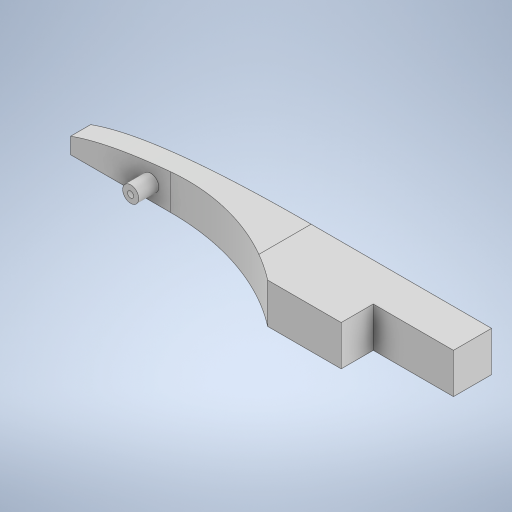
# Autodesk Inventor part: Norma
Saved by Autodesk Inventor 2023 (Build 270158000, 158)
## iProperties
Created: 2023-12-05
Part Number: Norma
Material: Všeobecné
Document SubType Name: Modeling
Designer: clu40164
Mass: 73.9819 g
Surface Area: 163.44 cm^2
Volume: 73.9819 cm^3
Density: 1 g/cm^3
Appearance: Výchozí
Author: clu40164
Autodesk Inventor part; units mm, degrees
ref_plane "YZ Plane" through (0, 0, 0) normal (1, 0, 0) x (0, 1, 0)
ref_plane "XZ Plane" through (0, 0, 0) normal (0, 1, 0) x (-1, 0, 0)
ref_plane "XY Plane" through (0, 0, 0) normal (0, 0, 1) x (1, 0, 0)
sketch "Náčrt1" plane through (0, 0, 0) normal (0, 0, 1) x (1, 0, 0)
  line L0 (0, 0) -> (200, 0)
  line L1 (200, 0) -> (200, 20)
  line L2 (200, 20) -> (110, 20)
  line L3 (0, 0) -> (0, 8)
  line L4 (0, 8) -> (32.9697, 20) construction
  line L5 (32.9697, 20) -> (110, 20) construction
  spline S0 degree 2 poles (0, 8) (32.9697, 20) (110, 20) knots 1 1 1 2 2 2
  dimension "d0" = 200
  dimension "d1" = 20
  dimension "d2" = 90
  dimension "d3" = 8
  dimension "d5" = 160
  constraints: 8 end point, 2 horizontal, 2 perpendicular, 1 vertical, 3 other
  measures "d0" distance of L0.start L0.end
  measures "d1" distance of L0.end L1.end
  measures "d2" distance of L1.end L2.end
  measures "d3" distance of L0.start L3.end
  measures "d5" angle of L5 L4
extrude "Vysunutí1" add sketch "Náčrt1" along normal blind 35
sketch "Náčrt2" plane through (0, 0, 0) normal (0, -1, 0) x (1, 0, 0)
  line L0 (0, 0) -> (0, 35) projected
  line L1 (0, 10) -> (50, 10)
  arc A0 (50, 10) -> (123.3144, 35) centre (50, 130) ccw
  line L2 (160, 35) -> (160, 19)
  line L3 (160, 19) -> (200, 19)
  line L4 (200, 0) -> (200, 35) projected
  line L5 (0, 35) -> (200, 35) projected
  line L6 (160, 35) -> (123.3144, 35)
  line L7 (200, 19) -> (200, 0)
  line L8 (0, 0) -> (200, 0) projected
  line L9 (0, 0) -> (0, 10)
  line L10 (0, 0) -> (200, 0)
  dimension "d8" = 50
  dimension "d9" = 240
  dimension "d11" = 16
  dimension "d12" = 40
  dimension "d13" = 10
  constraints: 14 end point, 5 perpendicular, 2 point on circle, 2 point on line, 1 centre point, 1 collinear, 1 horizontal, 1 horizontal alignment, 1 tangent, 1 vertical, 1 vertical alignment
  measures "d8" distance of L1.end L1.start
  measures "d9" diameter of A0
  measures "d11" distance of L2.start L2.end
  measures "d12" distance of L2.end L3.end
  measures "d13" distance of L0.start L1.start
extrude "Vysunutí2" cut sketch "Náčrt2" against normal blind 35 contours L0 L1 A0 L5 L2 L3 L4 L8 keep common part
sketch "Náčrt3" plane through (0, 0, 10) normal (0, 0, 1) x (1, 0, 0)
  circle A0 centre (40, 8) radius 4
  line L0 (0, 8) -> (0, 0) projected
  line L1 (0, 0) -> (50, 0) projected
  dimension "d16" = 8
  dimension "d17" = 40
  dimension "d18" = 8
  constraints: 1 centre point
  measures "d16" diameter of A0
  measures "d17" distance from line of A0.centre L0
  measures "d18" distance from line of L1 A0.centre
extrude "Vysunutí3" add sketch "Náčrt3" along normal blind 10
sketch "Náčrt4" plane through (40, 8, 20) normal (0, 0, 1) x (1, 0, 0)
  point P0 (-40, -8)
  point P1 (-0.0661, -0.1971)
hole "Díra1" at (39.9339, 7.8029, 20) direction (0, 0, -1) diameter 3 end through all
